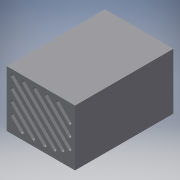
# Autodesk Inventor part: encolsure attempt 2
Saved by Autodesk Inventor 2019 (Build 230136000, 136)
## iProperties
Created: 2021-11-23
Part Number: encolsure attempt 2
Material: Generic
Document SubType Name: Modeling
Designer: Ian
Density: 1 g/cm^3
Appearance: Default
Author: Ian
Autodesk Inventor part; units mm, degrees
ref_plane "YZ Plane" through (0, 0, 0) normal (1, 0, 0) x (0, 1, 0)
ref_plane "XZ Plane" through (0, 0, 0) normal (0, 1, 0) x (-1, 0, 0)
ref_plane "XY Plane" through (0, 0, 0) normal (0, 0, 1) x (1, 0, 0)
sketch "Sketch1" plane through (0, 0, 0) normal (0, 0, 1) x (1, 0, 0)
  line L0 (13.1, 1.6) -> (6.35, 1.6) construction
  line L1 (13.1, 1.6) -> (13.1, 3.1) construction
  line L2 (6.35, 3.1) -> (13.1, 3.1) construction
  line L3 (6.35, 1.6) -> (6.35, 3.1) construction
  line L4 (0, 0) -> (17.3, 0) construction
  line L5 (17.3, 0) -> (17.3, 1.6) construction
  line L6 (0, 1.6) -> (17.3, 1.6) construction
  line L7 (0, 0) -> (0, 1.6) construction
  line L8 (-1, 0) -> (-1, 1.6) construction
  line L9 (0, 1.6) -> (-1, 1.6) construction
  line L10 (0, 0) -> (-1, 0) construction
  line L11 (18.3, 0) -> (17.3, 0) construction
  line L12 (18.3, 0) -> (18.3, 1.6) construction
  line L13 (18.3, 1.6) -> (17.3, 1.6) construction
  line L14 (14.65, 0) -> (14.65, 1.6) construction
  line L15 (17.15, 0) -> (17.15, 1.6) construction
  line L16 (-1, 3.1) -> (13.1, 3.1)
  line L17 (13.1, 3.1) -> (13.1, 1.6)
  line L18 (13.1, 1.6) -> (18.3, 1.6)
  line L19 (-1, 3.1) -> (-1, 0)
  line L20 (-1, 0) -> (18.3, 0)
  line L21 (18.3, 0) -> (18.3, 1.6)
  line L22 (-1, 1.6) -> (-1, 16.6)
  line L23 (-1, 16.6) -> (18.3, 16.6)
  line L24 (18.3, 16.6) -> (18.3, 1.6)
  line L25 (19.5, 0) -> (19.5, 17.8)
  line L26 (19.5, 17.8) -> (-2.2, 17.8)
  line L27 (-2.2, 17.8) -> (-2.2, 0)
  line L28 (-1, 0) -> (-2.2, 0)
  line L29 (18.3, 0) -> (19.5, 0)
  dimension "d1" = 15
  dimension "d2" = 1.2
  dimension "d4" = 1.2
  dimension "d5" = 1.2
  constraints: 32 end point, 5 collinear, 4 perpendicular, 2 point on line, 2 vertical, 1 horizontal, 4 other
  measures "d1" distance of L8.end L22.end
  measures "d2" distance between parallel lines of L23 L26
  measures "d4" distance between parallel lines of L24 L25
  measures "d5" distance between parallel lines of L22 L27
extrude "Extrusion1" add sketch "Sketch1" along normal blind 1.2
ref_plane "Work Plane1" through (-1, 0, -11.9) normal (-1, 0, 0) x (0, 0, 1)
sketch "Sketch2" plane through (-1, 0, -11.9) normal (-1, 0, 0) x (0, 0, 1)
  line L0 (11.9, 0) -> (-18.1, 0)
  line L1 (11.9, 17.8) -> (11.9, 0) projected
  line L2 (11.9, 17.8) -> (-18.1, 17.8)
  line L3 (-18.1, 17.8) -> (-18.1, 0)
  dimension "d8" = 30
  constraints: 6 end point, 2 horizontal, 1 perpendicular
  measures "d8" distance of L0.start L0.end
extrude "Extrusion2" add sketch "Sketch2" along normal blind 1.2
sketch "Sketch3" plane through (-2.2, 17.8, 1.2) normal (0, 1, 0) x (1, 0, 0)
  line L0 (0, 0) -> (21.7, 0) projected
  line L1 (0, 0) -> (21.7, 0)
  line L2 (21.7, 0) -> (21.7, 31.2)
  line L3 (21.7, 31.2) -> (0, 31.2)
  line L4 (0, 31.2) -> (0, 0)
  point P0 (2.2, 1.2)
  constraints: 8 end point, 2 parallel, 1 horizontal, 1 perpendicular
extrude "Extrusion3" add sketch "Sketch3" against normal blind 1.2
sketch "Sketch4" plane through (19.5, 0, 1.2) normal (1, 0, 0) x (0, 0, -1)
  line L0 (31.2, 17.8) -> (0, 17.8) projected
  line L1 (31.2, 0) -> (31.2, 16.6) projected
  line L2 (0, 17.8) -> (31.2, 17.8)
  line L3 (31.2, 17.8) -> (31.2, 0)
  line L4 (31.2, 0) -> (0, 0)
  line L5 (0, 0) -> (0, 17.8)
  point P0 (1.2, 0)
  constraints: 8 end point, 2 parallel, 1 horizontal, 1 perpendicular
extrude "Extrusion4" add sketch "Sketch4" against normal blind 1.2
sketch "Sketch5" plane through (19.5, 17.8, -30) normal (0, 0, -1) x (-1, 0, 0)
  line L0 (0, 0) -> (21.7, 0) projected
  line L1 (21.7, 0) -> (21.7, -17.8) projected
  line L2 (0, 0) -> (21.7, 0)
  line L3 (21.7, 0) -> (21.7, -17.8)
  line L4 (21.7, -17.8) -> (0, -17.8)
  line L5 (0, -17.8) -> (0, 0)
  point P0 (19.5, -17.8)
  constraints: 8 end point, 2 parallel, 1 horizontal, 1 perpendicular
extrude "Extrusion5" add sketch "Sketch5" against normal blind 1.2
sketch "Sketch6" plane through (-2.2, 0, 1.2) normal (0, -1, 0) x (1, 0, 0)
  line L0 (19.5, -14.1) -> (2.2, -14.1) construction
  line L1 (21.7, -31.2) -> (0, -31.2) projected
  line L2 (21.7, -31.2) -> (21.7, 0) projected
  line L3 (0, -31.2) -> (21.7, -31.2)
  line L4 (21.7, -31.2) -> (21.7, -14.1)
  line L5 (21.7, -14.1) -> (0, -14.1)
  line L6 (0, -14.1) -> (0, -31.2)
  point P0 (2.2, -1.2)
  constraints: 8 end point, 2 parallel, 1 collinear, 1 horizontal, 1 perpendicular, 1 point on line
extrude "Extrusion6" add sketch "Sketch6" against normal blind 1.2
sketch "Sketch7" plane through (0, 0, 0) normal (0, 0, -1) x (-1, 0, 0)
  line L0 (-13.1, 1.6) -> (-13.1, 3.1) construction
  line L1 (-17.3, 1.6) -> (0, 1.6) construction
  line L2 (-13.1, 3.1) -> (-6.35, 3.1) construction
  line L3 (-18.3, 16.6) -> (-18.3, 0) construction
  line L4 (1, 0) -> (-18.3, 0) construction
  line L5 (1, 0) -> (1, 16.6) construction
  line L6 (1, 16.6) -> (-18.3, 16.6) construction
  line L7 (-18.3, 1.6) -> (-14.1, 1.6)
  line L8 (-13.6, 2.1) -> (-13.6, 3.1)
  line L9 (-13.6, 3.1) -> (-18.3, 3.1)
  line L10 (-18.3, 3.1) -> (-18.3, 1.6)
  arc A0 (-14.1, 1.6) -> (-13.6, 2.1) centre (-14.1, 2.1) ccw
  point P0 (0, 0)
  dimension "d20" = 0.5
  dimension "d21" = 0.5
  constraints: 8 end point, 2 collinear, 2 parallel, 2 point on circle, 2 tangent, 1 centre point, 1 horizontal, 1 perpendicular, 1 point on line
  measures "d20" distance between parallel lines of L0 L8
  measures "d21" radius of A0
extrude "Extrusion7" add sketch "Sketch7" along normal blind 16.2
sketch "Sketch8" plane through (14.1, 1.6, 0) normal (0, -1, 0) x (1, 0, 0)
  circle A0 centre (1.8, -10.5) radius 1.25 projected
  circle A1 centre (1.8, -2.4) radius 1.25 projected
  circle A2 centre (1.8, -10.5) radius 0.975
  circle A3 centre (1.8, -2.4) radius 0.975
  point P0 (-14.1, 0)
  dimension "d24" = 1.95
  dimension "d25" = 1.95
  constraints: 2 centre point, 2 coincident
  measures "d24" diameter of A2
  measures "d25" diameter of A3
extrude "Extrusion8" cut sketch "Sketch8" against normal up to next contours A2 | A3
sketch "Sketch9" plane through (14.1, 1.6, 0) normal (0, -1, 0) x (1, 0, 0)
  circle A0 centre (1.8, -10.5) radius 0.975 projected
  circle A1 centre (1.8, -2.4) radius 0.975 projected
  line L0 (0, 0) -> (4.2, 0) projected
  line L1 (0, 0) -> (0, -16.2) projected
  line L2 (4.2, -16.2) -> (0, -16.2) projected
  line L3 (4.2, 0) -> (4.2, -16.2) projected
  line L4 (4.2, -12.9) -> (-15.1, -12.9) projected
  line L5 (-0.5, 0) -> (-0.5, -16.2) projected
  line L6 (4.2, -16.2) -> (0, -16.2) projected
  line L7 (-0.5, -16.2) -> (0, -16.2) projected
  line L8 (-0.5, 0) -> (-0.5, -16.2) projected
  line L9 (-0.5, -16.2) -> (4.2, -16.2) projected
  line L10 (-0.5, -12.9) -> (4.2, -12.9)
  line L11 (4.2, -12.9) -> (4.2, -16.2)
  line L12 (4.2, -16.2) -> (-0.5, -16.2)
  line L13 (-0.5, -16.2) -> (-0.5, -12.9)
  point P0 (-14.1, 0)
  constraints: 8 end point, 2 parallel, 2 point on line, 1 horizontal, 1 perpendicular
extrude "Extrusion9" add sketch "Sketch9" along normal blind 1.45 and the other way blind 1.35 contours L4 L3 L2 L1 | L1 L7 L5 L4
sketch "Sketch10" plane through (0, 0, 1.2) normal (0, 0, 1) x (1, 0, 0)
  line L0 (18.3, 16.6) -> (18.3, 3.1) construction
  line L1 (-1, 16.6) -> (18.3, 16.6) construction
  line L2 (-1, 0) -> (-1, 16.6) construction
  line L3 (0, 1.6) -> (17.3, 1.6) construction
  line L4 (18.3, 3.1) -> (13.6, 3.1) construction
  line L5 (13.6, 3.1) -> (13.6, 2.1) construction
  arc A0 (13.6, 2.1) -> (14.1, 1.6) centre (14.1, 2.1) ccw construction
  line L6 (0, 1.6) -> (-1, 1.6) construction
  line L7 (-1, 16.6) -> (14, 1.6) construction
  line L8 (2.6, 16.6) -> (17.6, 1.6) construction
  line L9 (6.2, 16.6) -> (21.2, 1.6) construction
  line L10 (9.8, 16.6) -> (24.8, 1.6) construction
  line L11 (13.4, 16.6) -> (28.4, 1.6) construction
  line L12 (-4.6, 16.6) -> (10.4, 1.6) construction
  line L13 (-1, 16.6) -> (14, 1.6) construction
  line L14 (2.6, 16.6) -> (17.6, 1.6) construction
  line L15 (6.2, 16.6) -> (21.2, 1.6) construction
  line L16 (9.8, 16.6) -> (24.8, 1.6) construction
  line L17 (-8.2, 16.6) -> (6.8, 1.6) construction
  line L18 (-4.6, 16.6) -> (10.4, 1.6) construction
  line L19 (-1, 16.6) -> (14, 1.6) construction
  line L20 (2.6, 16.6) -> (17.6, 1.6) construction
  line L21 (6.2, 16.6) -> (21.2, 1.6) construction
  line L22 (-11.8, 16.6) -> (3.2, 1.6) construction
  line L23 (-8.2, 16.6) -> (6.8, 1.6) construction
  line L24 (-4.6, 16.6) -> (10.4, 1.6) construction
  line L25 (-1, 16.6) -> (14, 1.6) construction
  line L26 (2.6, 16.6) -> (17.6, 1.6) construction
  arc A1 (17.2757, 11.8757) -> (18.1243, 12.7243) centre (17.7, 12.3) ccw
  arc A2 (14.4243, 16.4243) -> (13.5757, 15.5757) centre (14, 16) ccw
  arc A3 (17.2757, 8.2757) -> (18.1243, 9.1243) centre (17.7, 8.7) ccw
  arc A4 (10.8243, 16.4243) -> (9.9757, 15.5757) centre (10.4, 16) ccw
  line L27 (18.1243, 12.7243) -> (14.4243, 16.4243)
  line L28 (17.2757, 11.8757) -> (13.5757, 15.5757)
  line L29 (18.1243, 9.1243) -> (10.8243, 16.4243)
  line L30 (9.9757, 15.5757) -> (17.2757, 8.2757)
  arc A5 (7.2243, 16.4243) -> (6.3757, 15.5757) centre (6.8, 16) ccw
  arc A6 (3.6243, 16.4243) -> (2.7757, 15.5757) centre (3.2, 16) ccw
  arc A7 (0.0243, 16.4243) -> (-0.8243, 15.5757) centre (-0.4, 16) ccw
  arc A8 (0.0243, 12.8243) -> (-0.8243, 11.9757) centre (-0.4, 12.4) ccw
  arc A9 (0.0243, 9.2243) -> (-0.8243, 8.3757) centre (-0.4, 8.8) ccw
  arc A10 (0.0243, 5.6243) -> (-0.8243, 4.7757) centre (-0.4, 5.2) ccw
  arc A11 (2.1757, 1.7757) -> (3.0243, 2.6243) centre (2.6, 2.2) ccw
  arc A12 (5.7757, 1.7757) -> (6.6243, 2.6243) centre (6.2, 2.2) ccw
  arc A13 (9.3757, 1.7757) -> (10.2243, 2.6243) centre (9.8, 2.2) ccw
  arc A14 (12.5757, 2.1757) -> (13.4243, 3.0243) centre (13, 2.6) ccw
  arc A15 (15.0757, 3.2757) -> (15.9243, 4.1243) centre (15.5, 3.7) ccw
  arc A16 (17.2757, 4.6757) -> (18.1243, 5.5243) centre (17.7, 5.1) ccw
  line L31 (-0.8243, 4.7757) -> (2.1757, 1.7757)
  line L32 (0.0243, 5.6243) -> (3.0243, 2.6243)
  line L33 (-0.8243, 8.3757) -> (5.7757, 1.7757)
  line L34 (0.0243, 9.2243) -> (6.6243, 2.6243)
  line L35 (-0.8243, 11.9757) -> (9.3757, 1.7757)
  line L36 (10.2243, 2.6243) -> (0.0243, 12.8243)
  line L37 (-0.8243, 15.5757) -> (12.5757, 2.1757)
  line L38 (13.4243, 3.0243) -> (0.0243, 16.4243)
  line L39 (2.7757, 15.5757) -> (15.0757, 3.2757)
  line L40 (15.9243, 4.1243) -> (3.6243, 16.4243)
  line L41 (6.3757, 15.5757) -> (17.2757, 4.6757)
  line L42 (18.1243, 5.5243) -> (7.2243, 16.4243)
  point P0 (0, 0)
  dimension "d32" = 45
  dimension "d35" = 3.6
  dimension "d38" = 3.6
  dimension "d41" = 1.2
  dimension "d42" = 1.2
  dimension "d43" = 1.2
  dimension "d44" = 1.2
  dimension "d47" = 1.2
  dimension "d48" = 1.2
  dimension "d49" = 1.2
  dimension "d50" = 1.2
  dimension "d51" = 1.2
  dimension "d52" = 1.2
  dimension "d53" = 1.2
  dimension "d54" = 1.2
  dimension "d55" = 1.2
  dimension "d56" = 1.2
  dimension "d57" = 1.2
  dimension "d58" = 1.2
  constraints: 73 end point, 34 tangent, 32 point on circle, 17 point on line, 16 centre point, 12 parallel, 2 horizontal, 57 other
  measures "d32" angle of L1 L7
  measures "d35" distance of L1.start L8.start
  measures "d38" distance of L1.start L12.start
  measures "d41" diameter of A1
  measures "d42" diameter of A2
  measures "d43" diameter of A3
  measures "d44" diameter of A4
  measures "d47" diameter of A5
  measures "d48" diameter of A6
  measures "d49" diameter of A7
  measures "d50" diameter of A8
  measures "d51" diameter of A9
  measures "d52" diameter of A10
  measures "d53" diameter of A11
  measures "d54" diameter of A12
  measures "d55" diameter of A13
  measures "d56" diameter of A14
  measures "d57" diameter of A15
  measures "d58" diameter of A16
extrude "Extrusion10" cut sketch "Sketch10" against normal up to next
body "Solid1"
